Autodesk Fusion 360 part; units mm, degrees
(part 3 of 7)
  spline S37 degree 5 poles (-31.8463, 21.6348) (-31.8387, 21.6182) (-31.8236, 21.585) (-31.8007, 21.5353) (-31.7701, 21.4693) (-31.7314, 21.387) (-31.6925, 21.3049) (-31.6532, 21.2232) (-31.6135, 21.1418) (-31.5736, 21.0606) (-31.5333, 20.9798) (-31.4926, 20.8992) (-31.4516, 20.8189) (-31.4103, 20.739) (-31.3687, 20.6594) (-31.3267, 20.58) (-31.2844, 20.501) (-31.2417, 20.4223) (-31.1987, 20.3439) (-31.1553, 20.2659) (-31.1116, 20.1882) (-31.0676, 20.1108) (-31.0232, 20.0337) (-30.9785, 19.957) (-30.9334, 19.8806) (-30.888, 19.8046) (-30.8422, 19.7289) (-30.796, 19.6536) (-30.7496, 19.5787) (-30.7027, 19.5041) (-30.6555, 19.4299) (-30.608, 19.356) (-30.5601, 19.2825) (-30.5118, 19.2094) (-30.4631, 19.1368) (-30.4141, 19.0645) (-30.3647, 18.9925) (-30.315, 18.921) (-30.2649, 18.85) (-30.2144, 18.7793) (-30.1635, 18.709) (-30.1123, 18.6392) (-30.0606, 18.5699) (-30.0086, 18.5009) (-29.9561, 18.4325) (-29.9033, 18.3645) (-29.8501, 18.297) (-29.7965, 18.2299) (-29.7425, 18.1633) (-29.6881, 18.0972) (-29.6333, 18.0316) (-29.578, 17.9666) (-29.5222, 17.9021) (-29.466, 17.8383) (-29.4094, 17.775) (-29.3523, 17.7122) (-29.2948, 17.65) (-29.2369, 17.5883) (-29.1786, 17.5272) (-29.1198, 17.4666) (-29.0604, 17.4069) (-29.0004, 17.348) (-28.9396, 17.2901) (-28.8782, 17.2332) (-28.8162, 17.1772) (-28.7537, 17.1217) (-28.6909, 17.0668) (-28.6278, 17.0123) (-28.5642, 16.9585) (-28.4998, 16.906) (-28.434, 16.8556) (-28.3799, 16.8175) (-28.3382, 16.7905) (-28.3099, 16.7732) (-28.2957, 16.7647) knots -1 -1 -1 -1 -1 -1 -0.98571429 -0.97142857 -0.95714286 -0.94285714 -0.92857143 -0.91428571 -0.9 -0.88571429 -0.87142857 -0.85714286 -0.84285714 -0.82857143 -0.81428571 -0.8 -0.78571429 -0.77142857 -0.75714286 -0.74285714 -0.72857143 -0.71428571 -0.7 -0.68571429 -0.67142857 -0.65714286 -0.64285714 -0.62857143 -0.61428571 -0.6 -0.58571429 -0.57142857 -0.55714286 -0.54285714 -0.52857143 -0.51428571 -0.5 -0.48571429 -0.47142857 -0.45714286 -0.44285714 -0.42857143 -0.41428571 -0.4 -0.38571429 -0.37142857 -0.35714286 -0.34285714 -0.32857143 -0.31428571 -0.3 -0.28571429 -0.27142857 -0.25714286 -0.24285714 -0.22857143 -0.21428571 -0.2 -0.18571429 -0.17142857 -0.15714286 -0.14285714 -0.12857143 -0.11428571 -0.1 -0.08571429 -0.07142857 -0.05714286 -0.04285714 -0.02857143 -0.01428571 0 0 0 0 0 0
  line L37 (-28.2957, 16.7647) -> (-27.7863, 16.4626)
  arc A75 (-27.1922, 14.356) -> (-27.7863, 16.4626) centre (-28.5961, 15.0972) ccw
  arc A76 (-27.1922, 14.356) -> (-27.5975, 13.5607) centre (0, 0) ccw
  arc A77 (-29.6509, 12.8031) -> (-27.5975, 13.5607) centre (-29.0223, 14.2608) ccw
  line L38 (-29.6509, 12.8031) -> (-30.1947, 13.0376)
  spline S38 degree 5 poles (-30.1947, 13.0376) (-30.21, 13.0442) (-30.2406, 13.0569) (-30.2869, 13.0748) (-30.3496, 13.0962) (-30.429, 13.1197) (-30.5094, 13.141) (-30.5903, 13.1608) (-30.6714, 13.1798) (-30.7528, 13.1984) (-30.8344, 13.2163) (-30.9162, 13.2335) (-30.9983, 13.2498) (-31.0808, 13.2649) (-31.1637, 13.2788) (-31.247, 13.2917) (-31.3305, 13.3037) (-31.4142, 13.315) (-31.4982, 13.3255) (-31.5823, 13.3355) (-31.6666, 13.3448) (-31.7511, 13.3534) (-31.8359, 13.3614) (-31.9208, 13.3686) (-32.0059, 13.3751) (-32.0911, 13.3809) (-32.1766, 13.3861) (-32.2622, 13.3906) (-32.348, 13.3946) (-32.4339, 13.3979) (-32.52, 13.4007) (-32.6062, 13.4029) (-32.6925, 13.4045) (-32.779, 13.4055) (-32.8656, 13.4059) (-32.9523, 13.4058) (-33.0392, 13.4051) (-33.1262, 13.4038) (-33.2132, 13.4021) (-33.3004, 13.3997) (-33.3877, 13.3969) (-33.4751, 13.3935) (-33.5626, 13.3896) (-33.6502, 13.3852) (-33.7379, 13.3803) (-33.8257, 13.3748) (-33.9136, 13.3689) (-34.0016, 13.3624) (-34.0896, 13.3555) (-34.1778, 13.348) (-34.266, 13.3401) (-34.3542, 13.3317) (-34.4426, 13.3228) (-34.531, 13.3134) (-34.6195, 13.3035) (-34.7081, 13.2932) (-34.7967, 13.2824) (-34.8854, 13.2711) (-34.9741, 13.2594) (-35.063, 13.2472) (-35.1518, 13.2345) (-35.2407, 13.2214) (-35.3297, 13.2078) (-35.4187, 13.1938) (-35.5078, 13.1793) (-35.5969, 13.1644) (-35.686, 13.1491) (-35.7752, 13.1333) (-35.8644, 13.117) (-35.9537, 13.1003) (-36.043, 13.0832) (-36.1145, 13.0692) (-36.1681, 13.0584) (-36.2038, 13.0512) (-36.2217, 13.0476) knots 0 0 0 0 0 0 0.01428571 0.02857143 0.04285714 0.05714286 0.07142857 0.08571429 0.1 0.11428571 0.12857143 0.14285714 0.15714286 0.17142857 0.18571429 0.2 0.21428571 0.22857143 0.24285714 0.25714286 0.27142857 0.28571429 0.3 0.31428571 0.32857143 0.34285714 0.35714286 0.37142857 0.38571429 0.4 0.41428571 0.42857143 0.44285714 0.45714286 0.47142857 0.48571429 0.5 0.51428571 0.52857143 0.54285714 0.55714286 0.57142857 0.58571429 0.6 0.61428571 0.62857143 0.64285714 0.65714286 0.67142857 0.68571429 0.7 0.71428571 0.72857143 0.74285714 0.75714286 0.77142857 0.78571429 0.8 0.81428571 0.82857143 0.84285714 0.85714286 0.87142857 0.88571429 0.9 0.91428571 0.92857143 0.94285714 0.95714286 0.97142857 0.98571429 1 1 1 1 1 1
  arc A78 (-36.2217, 13.0476) -> (-36.9731, 10.7349) centre (0, 0) ccw
  spline S39 degree 5 poles (-36.9731, 10.7349) (-36.9608, 10.7214) (-36.9361, 10.6946) (-36.8991, 10.6544) (-36.8495, 10.601) (-36.7873, 10.5347) (-36.7249, 10.4687) (-36.6623, 10.4031) (-36.5994, 10.3379) (-36.5363, 10.2731) (-36.473, 10.2086) (-36.4095, 10.1446) (-36.3457, 10.0809) (-36.2817, 10.0176) (-36.2175, 9.9548) (-36.153, 9.8923) (-36.0883, 9.8302) (-36.0235, 9.7686) (-35.9583, 9.7073) (-35.893, 9.6465) (-35.8274, 9.5861) (-35.7616, 9.5261) (-35.6956, 9.4665) (-35.6293, 9.4074) (-35.5629, 9.3487) (-35.4962, 9.2904) (-35.4292, 9.2326) (-35.3621, 9.1752) (-35.2947, 9.1183) (-35.2271, 9.0618) (-35.1593, 9.0058) (-35.0912, 8.9503) (-35.023, 8.8952) (-34.9545, 8.8406) (-34.8857, 8.7865) (-34.8168, 8.7329) (-34.7476, 8.6798) (-34.6782, 8.6271) (-34.6086, 8.575) (-34.5387, 8.5234) (-34.4686, 8.4723) (-34.3983, 8.4218) (-34.3277, 8.3717) (-34.257, 8.3223) (-34.1859, 8.2734) (-34.1147, 8.225) (-34.0432, 8.1773) (-33.9715, 8.13) (-33.8996, 8.0834) (-33.8274, 8.0373) (-33.755, 7.9919) (-33.6823, 7.9471) (-33.6094, 7.9031) (-33.5362, 7.8597) (-33.4627, 7.817) (-33.389, 7.775) (-33.3151, 7.7336) (-33.241, 7.6928) (-33.1666, 7.6526) (-33.092, 7.6133) (-33.0171, 7.5748) (-32.9418, 7.5373) (-32.8662, 7.5011) (-32.7902, 7.4659) (-32.7139, 7.4318) (-32.6373, 7.3983) (-32.5606, 7.3655) (-32.4838, 7.3332) (-32.4067, 7.3017) (-32.3292, 7.2716) (-32.251, 7.244) (-32.1878, 7.2245) (-32.1398, 7.2117) (-32.1076, 7.204) (-32.0914, 7.2004) knots -1 -1 -1 -1 -1 -1 -0.98571429 -0.97142857 -0.95714286 -0.94285714 -0.92857143 -0.91428571 -0.9 -0.88571429 -0.87142857 -0.85714286 -0.84285714 -0.82857143 -0.81428571 -0.8 -0.78571429 -0.77142857 -0.75714286 -0.74285714 -0.72857143 -0.71428571 -0.7 -0.68571429 -0.67142857 -0.65714286 -0.64285714 -0.62857143 -0.61428571 -0.6 -0.58571429 -0.57142857 -0.55714286 -0.54285714 -0.52857143 -0.51428571 -0.5 -0.48571429 -0.47142857 -0.45714286 -0.44285714 -0.42857143 -0.41428571 -0.4 -0.38571429 -0.37142857 -0.35714286 -0.34285714 -0.32857143 -0.31428571 -0.3 -0.28571429 -0.27142857 -0.25714286 -0.24285714 -0.22857143 -0.21428571 -0.2 -0.18571429 -0.17142857 -0.15714286 -0.14285714 -0.12857143 -0.11428571 -0.1 -0.08571429 -0.07142857 -0.05714286 -0.04285714 -0.02857143 -0.01428571 0 0 0 0 0 0
  line L39 (-32.0914, 7.2004) -> (-31.5136, 7.0705)
  arc A79 (-30.2976, 5.2505) -> (-31.5136, 7.0705) centre (-31.8618, 5.5216) ccw
  circle A80 centre (0, 0) radius 7.5
  dimension "d9" = 15
  constraint coincident A0.centre A2.centre
  measures "d9" diameter of A80
extrude "Extruir3" add sketch "Boceto2 (2)" along normal blind 50 contours A80 bodies 1 in component "Spur Gear (20 teeth)"
sketch "Boceto3 (2)" plane through (0, 0, 63) normal (0, 0, 1) x (-1, 0, 0)
  circle A0 centre (0, 0) radius 7.5
  circle A1 centre (0, 0) radius 7.5
  constraint coincident A0.centre A1.centre
extrude "Extruir4" add sketch "Boceto3 (2)" along normal blind 15.297 bodies 1 in component "Spur Gear (20 teeth)"
sketch "Boceto4" plane through (0, 0, 78.297) normal (0, 0, 1) x (-1, 0, 0)
  circle A0 centre (0, 0) radius 7.5
  circle A1 centre (0, 0) radius 15
  dimension "d14" = 30
  constraint concentric A0 A1
  measures "d14" diameter of A1
extrude "Extruir1'" add sketch "Boceto4" along normal blind 2 separate body makes body 2
sketch "Boceto5" plane through (0, 0, 78.297) normal (0, 0, 1) x (-1, 0, 0)
  circle A0 centre (0, 0) radius 7.5
  circle A1 centre (0, 0) radius 7.5
  constraint coincident A0.centre A1.centre
extrude "Extruir2'" add sketch "Boceto5" along normal blind 2 bodies 2
sketch "Boceto6" plane through (0, 0, 80.297) normal (0, 0, 1) x (-1, 0, 0)
  circle A0 centre (0, 0) radius 15
  circle A1 centre (0, 12) radius 1
  circle A2 centre (-12, 0) radius 1
  circle A3 centre (12, 0) radius 1
  circle A4 centre (0, -12) radius 1
  dimension "d19" = 12
  dimension "d20" = 12
  dimension "d21" = 12
  dimension "d22" = 12
  dimension "d23" = 2
  dimension "d24" = 2
  dimension "d25" = 2
  dimension "d26" = 2
  measures "d19" distance of A0.centre A1.centre
  measures "d20" distance of A0.centre A2.centre
  measures "d21" distance of A0.centre A4.centre
  measures "d22" distance of A0.centre A3.centre
  measures "d23" diameter of A1
  measures "d24" diameter of A2
  measures "d25" diameter of A4
  measures "d26" diameter of A3
extrude "Extruir3'" cut sketch "Boceto6" against normal blind 2 contours A1 | A2 | A3 | A4 bodies 2
component "Spur Gear (20 teeth)" placed x (1, 0, 0) y (0, 1, 0) z (0, 0, 1) at (0, 0, 0)

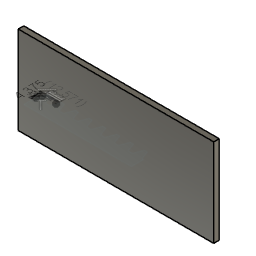
design "puerta mecatronica"
Autodesk Fusion 360 part; units mm, degrees
sketch "Boceto1" plane through (0, 0, 0) normal (0, 0, 1) x (1, 0, 0)
  line L0 (0, 0) -> (2.8663, 7.875)
  line L1 (0, 0) -> (64.0312, 0) construction
  line L2 (0, 0) -> (0, 4.375) construction
  line L3 (0, 4.375) -> (1.5924, 4.375) construction
  line L4 (1.5924, 4.375) -> (7.0924, 4.375) construction
  line L5 (7.0924, 4.375) -> (8.6847, 0)
  line L6 (7.0924, 4.375) -> (12.0861, 4.375) construction
  line L7 (7.0924, 4.375) -> (5.8185, 7.875)
  line L8 (7.0924, 4.375) -> (11.3868, 4.375) construction
  line L9 (5.8185, 7.875) -> (2.8663, 7.875)
  line L10 (8.6847, 0) -> (0, 0)
  dimension "d1" = 70
  dimension "d2" = 7.875
  dimension "d3" = 4.375
  dimension "d4" = 5.5
  dimension "d5" = 70
  dimension "d6" = 4.375
  dimension "d7" = 110
  dimension "d8" = 3.5
  constraint horizontal L1
  constraint coincident L0.start L1.start
  constraint perpendicular L1 L2
  constraint coincident L0 L3.end
  constraint perpendicular L2 L3
  constraint perpendicular L2 L4
  constraint horizontal L6
  constraint horizontal L8
  measures "d1" angle of L0 L1
  measures "d2" distance of L0.start L0.end
  measures "d3" distance of L0.start L2.end
  measures "d4" distance of L3.end L4.end
  measures "d5" angle of L5 L6
  measures "d6" distance of L4.end L5.end
  measures "d7" angle of L7 L8
  measures "d8" distance of L4.end L7.end
extrude "Extruir1" add sketch "Boceto1" along normal blind 13 makes body 1
pattern_linear "Patrón R1" count 8 spacing 12.5714 along (1, 0, 0) of "Extruir1" makes body 2 at (15.4663, 0, 8.6667) makes body 3 at (30.9327, 0, 8.6667) makes body 4 at (43.5041, 0, 4.3333) makes body 5 at (56.0755, 0, 4.3333) makes body 6 at (68.647, 0, 8.6667) makes body 7 at (81.2184, 0, 4.3333) makes body 8 at (93.7898, 0, 4.3333)
sketch "Boceto2" plane through (0, 0, 13) normal (0, 0, 1) x (-1, 0, 0)
  line L0 (-8.6847, 0) -> (-5.8185, -7.875)
  line L1 (-5.8185, -7.875) -> (-2.8663, -7.875)
  line L2 (-2.8663, -7.875) -> (0, 0)
  line L3 (0, 0) -> (-8.6847, 0)
  line L4 (0, 0) -> (-98, 0)
  line L5 (-98, 0) -> (-98, 16)
  line L6 (-98, 16) -> (0, 16)
  line L7 (0, 16) -> (0, 0)
  constraint horizontal L4
  constraint vertical L5
  constraint horizontal L6
  constraint vertical L7
  constraint coincident L2.end L3.start
extrude "Extruir2" add sketch "Boceto2" against normal blind 13 contours L3 L4 L5 L6 L7 bodies 1 2 3 4 5 6 7 8
fillet "Empalme1" radius 1.05 15 edges at (8.6847, 0, 6.5) (12.5714, 0, 6.5) (21.2562, 0, 6.5) (25.1429, 0, 6.5) (33.8276, 0, 6.5) (37.7143, 0, 6.5) (46.399, 0, 6.5) (50.2857, 0, 6.5) (58.9705, 0, 6.5) (62.8571, 0, 6.5) (71.5419, 0, 6.5) (75.4286, 0, 6.5) (84.1133, 0, 6.5) (88, 0, 6.5) (96.6847, 0, 6.5) on bodies 1
sketch "Boceto3" plane through (0, 0, 13) normal (0, 0, 1) x (-1, 0, 0)
  line L0 (-83.8619, -0.6909) -> (-81.247, -7.875)
  line L1 (-81.247, -7.875) -> (-78.2948, -7.875)
  line L2 (-78.2948, -7.875) -> (-75.68, -0.6909)
  arc A0 (-74.6934, 0) -> (-75.68, -0.6909) centre (-74.6934, -1.05) ccw
  line L3 (-74.6934, 0) -> (-72.2771, 0)
  arc A1 (-71.2904, -0.6909) -> (-72.2771, 0) centre (-72.2771, -1.05) ccw
  line L4 (-71.2904, -0.6909) -> (-68.6756, -7.875)
  line L5 (-68.6756, -7.875) -> (-65.7234, -7.875)
  line L6 (-65.7234, -7.875) -> (-63.1086, -0.6909)
  arc A2 (-62.1219, 0) -> (-63.1086, -0.6909) centre (-62.1219, -1.05) ccw
  line L7 (-62.1219, 0) -> (-59.7057, 0)
  arc A3 (-58.719, -0.6909) -> (-59.7057, 0) centre (-59.7057, -1.05) ccw
  line L8 (-58.719, -0.6909) -> (-56.1042, -7.875)
  line L9 (-56.1042, -7.875) -> (-53.152, -7.875)
  line L10 (-53.152, -7.875) -> (-50.5372, -0.6909)
  arc A4 (-49.5505, 0) -> (-50.5372, -0.6909) centre (-49.5505, -1.05) ccw
  line L11 (-49.5505, 0) -> (-47.1342, 0)
  arc A5 (-46.1476, -0.6909) -> (-47.1342, 0) centre (-47.1342, -1.05) ccw
  line L12 (-46.1476, -0.6909) -> (-43.5328, -7.875)
  line L13 (-43.5328, -7.875) -> (-40.5806, -7.875)
  line L14 (-40.5806, -7.875) -> (-37.9657, -0.6909)
  arc A6 (-36.9791, 0) -> (-37.9657, -0.6909) centre (-36.9791, -1.05) ccw
  line L15 (-36.9791, 0) -> (-34.5628, 0)
  arc A7 (-33.5761, -0.6909) -> (-34.5628, 0) centre (-34.5628, -1.05) ccw
  line L16 (-33.5761, -0.6909) -> (-30.9613, -7.875)
  line L17 (-30.9613, -7.875) -> (-28.0091, -7.875)
  line L18 (-28.0091, -7.875) -> (-25.3943, -0.6909)
  arc A8 (-24.4076, 0) -> (-25.3943, -0.6909) centre (-24.4076, -1.05) ccw
  line L19 (-24.4076, 0) -> (-21.9914, 0)
  arc A9 (-21.0047, -0.6909) -> (-21.9914, 0) centre (-21.9914, -1.05) ccw
  line L20 (-21.0047, -0.6909) -> (-18.3899, -7.875)
  line L21 (-18.3899, -7.875) -> (-15.4377, -7.875)
  line L22 (-15.4377, -7.875) -> (-12.8229, -0.6909)
  arc A10 (-11.8362, 0) -> (-12.8229, -0.6909) centre (-11.8362, -1.05) ccw
  line L23 (-11.8362, 0) -> (-9.42, 0)
  arc A11 (-8.4333, -0.6909) -> (-9.42, 0) centre (-9.42, -1.05) ccw
  line L24 (-8.4333, -0.6909) -> (-5.8185, -7.875)
  line L25 (-5.8185, -7.875) -> (-2.8663, -7.875)
  line L26 (-2.8663, -7.875) -> (0, 0)
  line L27 (0, 0) -> (0, 16)
  line L28 (0, 16) -> (-98, 16)
  line L29 (-98, 16) -> (-98, 0)
  line L30 (-98, 0) -> (-97.42, 0)
  arc A12 (-96.4333, -0.6909) -> (-97.42, 0) centre (-97.42, -1.05) ccw
  line L31 (-96.4333, -0.6909) -> (-93.8185, -7.875)
  line L32 (-93.8185, -7.875) -> (-90.8663, -7.875)
  line L33 (-90.8663, -7.875) -> (-88.2515, -0.6909)
  arc A13 (-87.2648, 0) -> (-88.2515, -0.6909) centre (-87.2648, -1.05) ccw
  line L34 (-87.2648, 0) -> (-84.8485, 0)
  arc A14 (-83.8619, -0.6909) -> (-84.8485, 0) centre (-84.8485, -1.05) ccw
  line L35 (0, 16) -> (-98, 16)
  line L36 (-98, 16) -> (-98, 11)
  line L37 (-98, 11) -> (0, 11)
  line L38 (0, 11) -> (0, 16)
  dimension "d19" = 5
  constraint horizontal L35
  constraint vertical L36
  constraint horizontal L37
  constraint vertical L38
  constraint coincident L29 L36.end
  constraint coincident L27.end L28.start
  measures "d19" distance of L27.end L37.end
extrude "Extruir3" add sketch "Boceto3" along normal blind 30 contours L27 L28 L29 L35 L36 L37 L38 bodies 1
sketch "Boceto4" plane through (0, 0, 0) normal (1, 0, 0) x (0, 1, 0)
sketch "Boceto5" plane through (0, 0, 0) normal (0, 0, -1) x (1, 0, 0)
  arc A0 (84.8485, 0) -> (83.8619, -0.6909) centre (84.8485, -1.05) ccw
  line L0 (84.8485, 0) -> (87.2648, 0)
  arc A1 (88.2515, -0.6909) -> (87.2648, 0) centre (87.2648, -1.05) ccw
  line L1 (88.2515, -0.6909) -> (90.8663, -7.875)
  line L2 (90.8663, -7.875) -> (93.8185, -7.875)
  line L3 (93.8185, -7.875) -> (96.4333, -0.6909)
  arc A2 (97.42, 0) -> (96.4333, -0.6909) centre (97.42, -1.05) ccw
  line L4 (97.42, 0) -> (98, 0)
  line L5 (98, 0) -> (98, 16)
  line L6 (98, 16) -> (0, 16)
  line L7 (0, 16) -> (0, 0)
  line L8 (0, 0) -> (2.8663, -7.875)
  line L9 (2.8663, -7.875) -> (5.8185, -7.875)
  line L10 (5.8185, -7.875) -> (8.4333, -0.6909)
  arc A3 (9.42, 0) -> (8.4333, -0.6909) centre (9.42, -1.05) ccw
  line L11 (9.42, 0) -> (11.8362, 0)
  arc A4 (12.8229, -0.6909) -> (11.8362, 0) centre (11.8362, -1.05) ccw
  line L12 (12.8229, -0.6909) -> (15.4377, -7.875)
  line L13 (15.4377, -7.875) -> (18.3899, -7.875)
  line L14 (18.3899, -7.875) -> (21.0047, -0.6909)
  arc A5 (21.9914, 0) -> (21.0047, -0.6909) centre (21.9914, -1.05) ccw
  line L15 (21.9914, 0) -> (24.4076, 0)
  arc A6 (25.3943, -0.6909) -> (24.4076, 0) centre (24.4076, -1.05) ccw
  line L16 (25.3943, -0.6909) -> (28.0091, -7.875)
  line L17 (28.0091, -7.875) -> (30.9613, -7.875)
  line L18 (30.9613, -7.875) -> (33.5761, -0.6909)
  arc A7 (34.5628, 0) -> (33.5761, -0.6909) centre (34.5628, -1.05) ccw
  line L19 (34.5628, 0) -> (36.9791, 0)
  arc A8 (37.9657, -0.6909) -> (36.9791, 0) centre (36.9791, -1.05) ccw
  line L20 (37.9657, -0.6909) -> (40.5806, -7.875)
  line L21 (40.5806, -7.875) -> (43.5328, -7.875)
  line L22 (43.5328, -7.875) -> (46.1476, -0.6909)
  arc A9 (47.1342, 0) -> (46.1476, -0.6909) centre (47.1342, -1.05) ccw
  line L23 (47.1342, 0) -> (49.5505, 0)
  arc A10 (50.5372, -0.6909) -> (49.5505, 0) centre (49.5505, -1.05) ccw
  line L24 (50.5372, -0.6909) -> (53.152, -7.875)
  line L25 (53.152, -7.875) -> (56.1042, -7.875)
  line L26 (56.1042, -7.875) -> (58.719, -0.6909)
  arc A11 (59.7057, 0) -> (58.719, -0.6909) centre (59.7057, -1.05) ccw
  line L27 (59.7057, 0) -> (62.1219, 0)
  arc A12 (63.1086, -0.6909) -> (62.1219, 0) centre (62.1219, -1.05) ccw
  line L28 (63.1086, -0.6909) -> (65.7234, -7.875)
  line L29 (65.7234, -7.875) -> (68.6756, -7.875)
  line L30 (68.6756, -7.875) -> (71.2904, -0.6909)
  arc A13 (72.2771, 0) -> (71.2904, -0.6909) centre (72.2771, -1.05) ccw
  line L31 (72.2771, 0) -> (74.6934, 0)
  arc A14 (75.68, -0.6909) -> (74.6934, 0) centre (74.6934, -1.05) ccw
  line L32 (75.68, -0.6909) -> (78.2948, -7.875)
  line L33 (78.2948, -7.875) -> (81.247, -7.875)
  line L34 (81.247, -7.875) -> (83.8619, -0.6909)
  line L35 (98, 16) -> (0, 16)
  line L36 (0, 16) -> (0, 11)
  line L37 (0, 11) -> (98, 11)
  line L38 (98, 11) -> (98, 16)
  constraint horizontal L35
  constraint vertical L36
  constraint horizontal L37
  constraint vertical L38
  constraint coincident L7 L36.end
  constraint coincident L5.end L6.start
extrude "Extruir4" add sketch "Boceto5" along normal blind 5 contours L5 L6 L7 L35 L36 L37 L38 bodies 1
sketch "Boceto6" plane through (0, 0, 43) normal (0, 0, 1) x (-1, 0, 0)
  line L0 (0, 11) -> (0, 16)
  line L1 (0, 16) -> (-98, 16)
  line L2 (-98, 16) -> (-98, 11)
  line L3 (-98, 11) -> (0, 11)
  line L4 (0, 16) -> (-98, 16)
  line L5 (-98, 16) -> (-98, 11)
  line L6 (-98, 11) -> (0, 11)
  line L7 (0, 11) -> (0, 16)
  constraint horizontal L4
  constraint vertical L5
  constraint horizontal L6
  constraint vertical L7
  constraint coincident L2.end L3.start
  constraint coincident L0.end L1.start
extrude "Extruir5" add sketch "Boceto6" along normal blind 32 bodies 1
sketch "Boceto7" plane through (98, 0, 0) normal (1, 0, 0) x (0, 1, 0)
  line L0 (0, 13) -> (-11, 13)
  line L1 (-11, 13) -> (-11, 75)
  line L2 (-11, 75) -> (-16, 75)
  line L3 (-16, 75) -> (-16, -5)
  line L4 (-16, -5) -> (-11, -5)
  line L5 (-11, -5) -> (-11, 0)
  line L6 (-11, 0) -> (0, 0)
  line L7 (0, 0) -> (0, 13)
  line L8 (-11, 75) -> (-16, 75)
  line L9 (-16, 75) -> (-16, -5)
  line L10 (-16, -5) -> (-11, -5)
  line L11 (-11, -5) -> (-11, 75)
  constraint horizontal L8
  constraint vertical L9
  constraint horizontal L10
  constraint vertical L11
  constraint coincident L3.end L4.start
  constraint coincident L1.end L2.start
extrude "Extruir6" add sketch "Boceto7" along normal blind 80 contours L1 L2 L3 L4 L5 L8 L9 L10 L11 bodies 1
sketch "Boceto8" plane through (0, 0, 13) normal (0, 0, 1) x (-1, 0, 0)
  line L0 (0, 11) -> (-98, 11)
  line L1 (-98, 11) -> (-98, 0)
  line L2 (-98, 0) -> (-97.42, 0)
  arc A0 (-96.4333, -0.6909) -> (-97.42, 0) centre (-97.42, -1.05) ccw
  line L3 (-96.4333, -0.6909) -> (-93.8185, -7.875)
  line L4 (-93.8185, -7.875) -> (-90.8663, -7.875)
  line L5 (-90.8663, -7.875) -> (-88.2515, -0.6909)
  arc A1 (-87.2648, 0) -> (-88.2515, -0.6909) centre (-87.2648, -1.05) ccw
  line L6 (-87.2648, 0) -> (-84.8485, 0)
  arc A2 (-83.8619, -0.6909) -> (-84.8485, 0) centre (-84.8485, -1.05) ccw
  line L7 (-83.8619, -0.6909) -> (-81.247, -7.875)
  line L8 (-81.247, -7.875) -> (-78.2948, -7.875)
  line L9 (-78.2948, -7.875) -> (-75.68, -0.6909)
  arc A3 (-74.6934, 0) -> (-75.68, -0.6909) centre (-74.6934, -1.05) ccw
  line L10 (-74.6934, 0) -> (-72.2771, 0)
  arc A4 (-71.2904, -0.6909) -> (-72.2771, 0) centre (-72.2771, -1.05) ccw
  line L11 (-71.2904, -0.6909) -> (-68.6756, -7.875)
  line L12 (-68.6756, -7.875) -> (-65.7234, -7.875)
  line L13 (-65.7234, -7.875) -> (-63.1086, -0.6909)
  arc A5 (-62.1219, 0) -> (-63.1086, -0.6909) centre (-62.1219, -1.05) ccw
  line L14 (-62.1219, 0) -> (-59.7057, 0)
  arc A6 (-58.719, -0.6909) -> (-59.7057, 0) centre (-59.7057, -1.05) ccw
  line L15 (-58.719, -0.6909) -> (-56.1042, -7.875)
  line L16 (-56.1042, -7.875) -> (-53.152, -7.875)
  line L17 (-53.152, -7.875) -> (-50.5372, -0.6909)
  arc A7 (-49.5505, 0) -> (-50.5372, -0.6909) centre (-49.5505, -1.05) ccw
  line L18 (-49.5505, 0) -> (-47.1342, 0)
  arc A8 (-46.1476, -0.6909) -> (-47.1342, 0) centre (-47.1342, -1.05) ccw
  line L19 (-46.1476, -0.6909) -> (-43.5328, -7.875)
  line L20 (-43.5328, -7.875) -> (-40.5806, -7.875)
  line L21 (-40.5806, -7.875) -> (-37.9657, -0.6909)
  arc A9 (-36.9791, 0) -> (-37.9657, -0.6909) centre (-36.9791, -1.05) ccw
  line L22 (-36.9791, 0) -> (-34.5628, 0)
  arc A10 (-33.5761, -0.6909) -> (-34.5628, 0) centre (-34.5628, -1.05) ccw
  line L23 (-33.5761, -0.6909) -> (-30.9613, -7.875)
  line L24 (-30.9613, -7.875) -> (-28.0091, -7.875)
  line L25 (-28.0091, -7.875) -> (-25.3943, -0.6909)
  arc A11 (-24.4076, 0) -> (-25.3943, -0.6909) centre (-24.4076, -1.05) ccw
  line L26 (-24.4076, 0) -> (-21.9914, 0)
  arc A12 (-21.0047, -0.6909) -> (-21.9914, 0) centre (-21.9914, -1.05) ccw
  line L27 (-21.0047, -0.6909) -> (-18.3899, -7.875)
  line L28 (-18.3899, -7.875) -> (-15.4377, -7.875)
  line L29 (-15.4377, -7.875) -> (-12.8229, -0.6909)
  arc A13 (-11.8362, 0) -> (-12.8229, -0.6909) centre (-11.8362, -1.05) ccw
  line L30 (-11.8362, 0) -> (-9.42, 0)
  arc A14 (-8.4333, -0.6909) -> (-9.42, 0) centre (-9.42, -1.05) ccw
  line L31 (-8.4333, -0.6909) -> (-5.8185, -7.875)
  line L32 (-5.8185, -7.875) -> (-2.8663, -7.875)
  line L33 (-2.8663, -7.875) -> (0, 0)
  line L34 (0, 0) -> (0, 11)
  line L35 (0, 0) -> (0, -4.375) construction
  line L36 (0, -4.375) -> (-1.5924, -4.375) construction
  line L37 (-1.5924, -4.375) -> (-14.1638, -4.375) construction
  dimension "d28" = 4.375
  dimension "d29" = 12.5714
  constraint coincident L33.end L34.start
  constraint parallel L34 L35
  constraint coincident L33 L36.end
  constraint perpendicular L35 L36
  constraint coincident L29 L37.end
  constraint horizontal L37
  measures "d28" distance of L33.end L35.end
  measures "d29" distance of L36.end L37.end

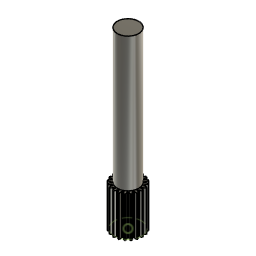
design "engranaje mecatronica"
part number: arrangementsContainer
description: Spur Gear; Module: 0.5; Num Teeth: 20; Pressure Angle: 20.0; Backlash: 0.00 mm
Autodesk Fusion 360 part; units mm, degrees
sketch "Boceto1" plane through (0, 0, 0) normal (0, 0, 1) x (1, 0, 0) in component "Spur Gear (20 teeth)"
  circle A0 centre (0, 0) radius 4.3492
extrude "Extruir1" add sketch "Boceto1" along normal blind 15 in component "Spur Gear (20 teeth)"
sketch "Boceto2" plane through (0, 0, 0) normal (0, 0, 1) x (1, 0, 0) in component "Spur Gear (20 teeth)"
  spline S0 degree 5 poles (4.678, -0.4384) (4.6803, -0.4386) (4.6849, -0.439) (4.6919, -0.4393) (4.7012, -0.4395) (4.7128, -0.4392) (4.7245, -0.4386) (4.7361, -0.4378) (4.7478, -0.4368) (4.7595, -0.4357) (4.7712, -0.4346) (4.7829, -0.4334) (4.7947, -0.432) (4.8064, -0.4304) (4.8181, -0.4287) (4.8299, -0.4269) (4.8416, -0.4248) (4.8534, -0.4227) (4.8651, -0.4205) (4.8769, -0.4182) (4.8886, -0.4158) (4.9004, -0.4133) (4.9122, -0.4106) (4.9239, -0.4079) (4.9357, -0.4051) (4.9475, -0.4022) (4.9593, -0.3991) (4.971, -0.396) (4.9828, -0.3928) (4.9946, -0.3895) (5.0064, -0.3861) (5.0181, -0.3826) (5.0299, -0.3791) (5.0417, -0.3754) (5.0535, -0.3717) (5.0652, -0.3679) (5.077, -0.364) (5.0888, -0.36) (5.1005, -0.3559) (5.1123, -0.3518) (5.124, -0.3476) (5.1358, -0.3433) (5.1475, -0.3389) (5.1593, -0.3344) (5.171, -0.3299) (5.1828, -0.3253) (5.1945, -0.3206) (5.2062, -0.3158) (5.2179, -0.311) (5.2297, -0.3061) (5.2414, -0.3011) (5.2531, -0.296) (5.2648, -0.2909) (5.2765, -0.2857) (5.2882, -0.2804) (5.2998, -0.2751) (5.3115, -0.2697) (5.3232, -0.2642) (5.3348, -0.2586) (5.3465, -0.253) (5.3581, -0.2473) (5.3698, -0.2415) (5.3814, -0.2357) (5.393, -0.2298) (5.4047, -0.2238) (5.4163, -0.2178) (5.4279, -0.2117) (5.4395, -0.2055) (5.451, -0.1993) (5.4626, -0.193) (5.4742, -0.1866) (5.4834, -0.1815) (5.4903, -0.1776) (5.4949, -0.175) (5.4973, -0.1737) knots 0 0 0 0 0 0 0.01428571 0.02857143 0.04285714 0.05714286 0.07142857 0.08571429 0.1 0.11428571 0.12857143 0.14285714 0.15714286 0.17142857 0.18571429 0.2 0.21428571 0.22857143 0.24285714 0.25714286 0.27142857 0.28571429 0.3 0.31428571 0.32857143 0.34285714 0.35714286 0.37142857 0.38571429 0.4 0.41428571 0.42857143 0.44285714 0.45714286 0.47142857 0.48571429 0.5 0.51428571 0.52857143 0.54285714 0.55714286 0.57142857 0.58571429 0.6 0.61428571 0.62857143 0.64285714 0.65714286 0.67142857 0.68571429 0.7 0.71428571 0.72857143 0.74285714 0.75714286 0.77142857 0.78571429 0.8 0.81428571 0.82857143 0.84285714 0.85714286 0.87142857 0.88571429 0.9 0.91428571 0.92857143 0.94285714 0.95714286 0.97142857 0.98571429 1 1 1 1 1 1
  spline S1 degree 5 poles (4.678, 0.4384) (4.6803, 0.4386) (4.6849, 0.439) (4.6919, 0.4393) (4.7012, 0.4395) (4.7128, 0.4392) (4.7245, 0.4386) (4.7361, 0.4378) (4.7478, 0.4368) (4.7595, 0.4357) (4.7712, 0.4346) (4.7829, 0.4334) (4.7947, 0.432) (4.8064, 0.4304) (4.8181, 0.4287) (4.8299, 0.4269) (4.8416, 0.4248) (4.8534, 0.4227) (4.8651, 0.4205) (4.8769, 0.4182) (4.8886, 0.4158) (4.9004, 0.4133) (4.9122, 0.4106) (4.9239, 0.4079) (4.9357, 0.4051) (4.9475, 0.4022) (4.9593, 0.3991) (4.971, 0.396) (4.9828, 0.3928) (4.9946, 0.3895) (5.0064, 0.3861) (5.0181, 0.3826) (5.0299, 0.3791) (5.0417, 0.3754) (5.0535, 0.3717) (5.0652, 0.3679) (5.077, 0.364) (5.0888, 0.36) (5.1005, 0.3559) (5.1123, 0.3518) (5.124, 0.3476) (5.1358, 0.3433) (5.1475, 0.3389) (5.1593, 0.3344) (5.171, 0.3299) (5.1828, 0.3253) (5.1945, 0.3206) (5.2062, 0.3158) (5.2179, 0.311) (5.2297, 0.3061) (5.2414, 0.3011) (5.2531, 0.296) (5.2648, 0.2909) (5.2765, 0.2857) (5.2882, 0.2804) (5.2998, 0.2751) (5.3115, 0.2697) (5.3232, 0.2642) (5.3348, 0.2586) (5.3465, 0.253) (5.3581, 0.2473) (5.3698, 0.2415) (5.3814, 0.2357) (5.393, 0.2298) (5.4047, 0.2238) (5.4163, 0.2178) (5.4279, 0.2117) (5.4395, 0.2055) (5.451, 0.1993) (5.4626, 0.193) (5.4742, 0.1866) (5.4834, 0.1815) (5.4903, 0.1776) (5.4949, 0.175) (5.4973, 0.1737) knots 0 0 0 0 0 0 0.01428571 0.02857143 0.04285714 0.05714286 0.07142857 0.08571429 0.1 0.11428571 0.12857143 0.14285714 0.15714286 0.17142857 0.18571429 0.2 0.21428571 0.22857143 0.24285714 0.25714286 0.27142857 0.28571429 0.3 0.31428571 0.32857143 0.34285714 0.35714286 0.37142857 0.38571429 0.4 0.41428571 0.42857143 0.44285714 0.45714286 0.47142857 0.48571429 0.5 0.51428571 0.52857143 0.54285714 0.55714286 0.57142857 0.58571429 0.6 0.61428571 0.62857143 0.64285714 0.65714286 0.67142857 0.68571429 0.7 0.71428571 0.72857143 0.74285714 0.75714286 0.77142857 0.78571429 0.8 0.81428571 0.82857143 0.84285714 0.85714286 0.87142857 0.88571429 0.9 0.91428571 0.92857143 0.94285714 0.95714286 0.97142857 0.98571429 1 1 1 1 1 1
  arc A0 (5.4973, -0.1737) -> (5.4973, 0.1737) centre (0, 0) ccw
  line L0 (4.3203, -0.4058) -> (4.678, -0.4384)
  line L1 (4.3203, 0.4058) -> (4.678, 0.4384)
  line L2 (4.3203, -0.4058) -> (4.3203, 0.4058)
  point P0 (4.7355, -0.4378)
  point P1 (4.7935, -0.4321)
  point P2 (4.8518, -0.423)
  point P3 (4.9103, -0.411)
  point P4 (4.9689, -0.3966)
  point P5 (5.0277, -0.3798)
  point P6 (5.0865, -0.3608)
  point P7 (5.1453, -0.3397)
  point P8 (5.2041, -0.3167)
  point P9 (5.2629, -0.2917)
  point P10 (5.3217, -0.2649)
  point P11 (5.3803, -0.2363)
  point P12 (5.4389, -0.2058)
  point P13 (4.7355, 0.4378)
  point P14 (4.7935, 0.4321)
  point P15 (4.8518, 0.423)
  point P16 (4.9103, 0.411)
  point P17 (4.9689, 0.3966)
  point P18 (5.0277, 0.3798)
  point P19 (5.0865, 0.3608)
  point P20 (5.1453, 0.3397)
  point P21 (5.2041, 0.3167)
  point P22 (5.2629, 0.2917)
  point P23 (5.3217, 0.2649)
  point P24 (5.3803, 0.2363)
  point P25 (5.4389, 0.2058)
extrude "Extruir2" add sketch "Boceto2" along normal blind 15 in component "Spur Gear (20 teeth)"
fillet "Empalme1" radius 0.1 2 edges at (4.3301, -0.4067, 7.5) (4.3301, 0.4067, 7.5) in component "Spur Gear (20 teeth)"
pattern_circular "Patrón C1" count 20 over 360 about axis through (0, 0, 0) along (0, 0, 1) of "Extruir2", "Empalme1" in component "Spur Gear (20 teeth)"
sketch "Boceto3" plane through (0, 0, 0) normal (0, 0, 1) x (1, 0, 0) in component "Spur Gear (20 teeth)"
  circle A0 centre (0, 0) radius 5 construction
sketch "Boceto1 (2)" plane through (0, 0, 15) normal (0, 0, 1) x (-1, 0, 0)
  arc A0 (-4.2641, 0.8559) -> (-4.3199, 0.5037) centre (0, 0) ccw
  arc A1 (-4.4283, 0.4157) -> (-4.3199, 0.5037) centre (-4.4193, 0.5152) ccw
  line L0 (-4.4283, 0.4157) -> (-4.678, 0.4384)
  spline S0 degree 5 poles (-4.678, 0.4384) (-4.6803, 0.4386) (-4.6849, 0.439) (-4.6919, 0.4393) (-4.7012, 0.4395) (-4.7128, 0.4392) (-4.7245, 0.4386) (-4.7361, 0.4378) (-4.7478, 0.4368) (-4.7595, 0.4357) (-4.7712, 0.4346) (-4.7829, 0.4334) (-4.7947, 0.432) (-4.8064, 0.4304) (-4.8181, 0.4287) (-4.8299, 0.4269) (-4.8416, 0.4248) (-4.8534, 0.4227) (-4.8651, 0.4205) (-4.8769, 0.4182) (-4.8886, 0.4158) (-4.9004, 0.4133) (-4.9122, 0.4106) (-4.9239, 0.4079) (-4.9357, 0.4051) (-4.9475, 0.4022) (-4.9593, 0.3991) (-4.971, 0.396) (-4.9828, 0.3928) (-4.9946, 0.3895) (-5.0064, 0.3861) (-5.0181, 0.3826) (-5.0299, 0.3791) (-5.0417, 0.3754) (-5.0535, 0.3717) (-5.0652, 0.3679) (-5.077, 0.364) (-5.0888, 0.36) (-5.1005, 0.3559) (-5.1123, 0.3518) (-5.124, 0.3476) (-5.1358, 0.3433) (-5.1475, 0.3389) (-5.1593, 0.3344) (-5.171, 0.3299) (-5.1828, 0.3253) (-5.1945, 0.3206) (-5.2062, 0.3158) (-5.2179, 0.311) (-5.2297, 0.3061) (-5.2414, 0.3011) (-5.2531, 0.296) (-5.2648, 0.2909) (-5.2765, 0.2857) (-5.2882, 0.2804) (-5.2998, 0.2751) (-5.3115, 0.2697) (-5.3232, 0.2642) (-5.3348, 0.2586) (-5.3465, 0.253) (-5.3581, 0.2473) (-5.3698, 0.2415) (-5.3814, 0.2357) (-5.393, 0.2298) (-5.4047, 0.2238) (-5.4163, 0.2178) (-5.4279, 0.2117) (-5.4395, 0.2055) (-5.451, 0.1993) (-5.4626, 0.193) (-5.4742, 0.1866) (-5.4834, 0.1815) (-5.4903, 0.1776) (-5.4949, 0.175) (-5.4973, 0.1737) knots 0 0 0 0 0 0 0.01428571 0.02857143 0.04285714 0.05714286 0.07142857 0.08571429 0.1 0.11428571 0.12857143 0.14285714 0.15714286 0.17142857 0.18571429 0.2 0.21428571 0.22857143 0.24285714 0.25714286 0.27142857 0.28571429 0.3 0.31428571 0.32857143 0.34285714 0.35714286 0.37142857 0.38571429 0.4 0.41428571 0.42857143 0.44285714 0.45714286 0.47142857 0.48571429 0.5 0.51428571 0.52857143 0.54285714 0.55714286 0.57142857 0.58571429 0.6 0.61428571 0.62857143 0.64285714 0.65714286 0.67142857 0.68571429 0.7 0.71428571 0.72857143 0.74285714 0.75714286 0.77142857 0.78571429 0.8 0.81428571 0.82857143 0.84285714 0.85714286 0.87142857 0.88571429 0.9 0.91428571 0.92857143 0.94285714 0.95714286 0.97142857 0.98571429 1 1 1 1 1 1
  arc A2 (-5.4973, 0.1737) -> (-5.4973, -0.1737) centre (0, 0) ccw
  spline S1 degree 5 poles (-5.4973, -0.1737) (-5.4949, -0.175) (-5.4903, -0.1776) (-5.4834, -0.1815) (-5.4742, -0.1866) (-5.4626, -0.193) (-5.451, -0.1993) (-5.4395, -0.2055) (-5.4279, -0.2117) (-5.4163, -0.2178) (-5.4047, -0.2238) (-5.393, -0.2298) (-5.3814, -0.2357) (-5.3698, -0.2415) (-5.3581, -0.2473) (-5.3465, -0.253) (-5.3348, -0.2586) (-5.3232, -0.2642) (-5.3115, -0.2697) (-5.2998, -0.2751) (-5.2882, -0.2804) (-5.2765, -0.2857) (-5.2648, -0.2909) (-5.2531, -0.296) (-5.2414, -0.3011) (-5.2297, -0.3061) (-5.2179, -0.311) (-5.2062, -0.3158) (-5.1945, -0.3206) (-5.1828, -0.3253) (-5.171, -0.3299) (-5.1593, -0.3344) (-5.1475, -0.3389) (-5.1358, -0.3433) (-5.124, -0.3476) (-5.1123, -0.3518) (-5.1005, -0.3559) (-5.0888, -0.36) (-5.077, -0.364) (-5.0652, -0.3679) (-5.0535, -0.3717) (-5.0417, -0.3754) (-5.0299, -0.3791) (-5.0181, -0.3826) (-5.0064, -0.3861) (-4.9946, -0.3895) (-4.9828, -0.3928) (-4.971, -0.396) (-4.9593, -0.3991) (-4.9475, -0.4022) (-4.9357, -0.4051) (-4.9239, -0.4079) (-4.9122, -0.4106) (-4.9004, -0.4133) (-4.8886, -0.4158) (-4.8769, -0.4182) (-4.8651, -0.4205) (-4.8534, -0.4227) (-4.8416, -0.4248) (-4.8299, -0.4269) (-4.8181, -0.4287) (-4.8064, -0.4304) (-4.7947, -0.432) (-4.7829, -0.4334) (-4.7712, -0.4346) (-4.7595, -0.4357) (-4.7478, -0.4368) (-4.7361, -0.4378) (-4.7245, -0.4386) (-4.7128, -0.4392) (-4.7012, -0.4395) (-4.6919, -0.4393) (-4.6849, -0.439) (-4.6803, -0.4386) (-4.678, -0.4384) knots -1 -1 -1 -1 -1 -1 -0.98571429 -0.97142857 -0.95714286 -0.94285714 -0.92857143 -0.91428571 -0.9 -0.88571429 -0.87142857 -0.85714286 -0.84285714 -0.82857143 -0.81428571 -0.8 -0.78571429 -0.77142857 -0.75714286 -0.74285714 -0.72857143 -0.71428571 -0.7 -0.68571429 -0.67142857 -0.65714286 -0.64285714 -0.62857143 -0.61428571 -0.6 -0.58571429 -0.57142857 -0.55714286 -0.54285714 -0.52857143 -0.51428571 -0.5 -0.48571429 -0.47142857 -0.45714286 -0.44285714 -0.42857143 -0.41428571 -0.4 -0.38571429 -0.37142857 -0.35714286 -0.34285714 -0.32857143 -0.31428571 -0.3 -0.28571429 -0.27142857 -0.25714286 -0.24285714 -0.22857143 -0.21428571 -0.2 -0.18571429 -0.17142857 -0.15714286 -0.14285714 -0.12857143 -0.11428571 -0.1 -0.08571429 -0.07142857 -0.05714286 -0.04285714 -0.02857143 -0.01428571 0 0 0 0 0 0
  line L1 (-4.678, -0.4384) -> (-4.4283, -0.4157)
  arc A3 (-4.3199, -0.5037) -> (-4.4283, -0.4157) centre (-4.4193, -0.5152) ccw
  arc A4 (-4.3199, -0.5037) -> (-4.2641, -0.8559) centre (0, 0) ccw
  arc A5 (-4.34, -0.9731) -> (-4.2641, -0.8559) centre (-4.3622, -0.8756) ccw
  line L2 (-4.34, -0.9731) -> (-4.5845, -1.0286)
  spline S2 degree 5 poles (-4.5845, -1.0286) (-4.5868, -1.0291) (-4.5913, -1.0302) (-4.598, -1.032) (-4.6069, -1.0348) (-4.6179, -1.0386) (-4.6288, -1.0428) (-4.6396, -1.0472) (-4.6504, -1.0517) (-4.6612, -1.0564) (-4.672, -1.061) (-4.6828, -1.0659) (-4.6935, -1.0708) (-4.7042, -1.0759) (-4.7148, -1.0811) (-4.7254, -1.0865) (-4.7359, -1.0921) (-4.7465, -1.0977) (-4.7569, -1.1035) (-4.7674, -1.1093) (-4.7779, -1.1153) (-4.7883, -1.1213) (-4.7987, -1.1274) (-4.809, -1.1336) (-4.8193, -1.14) (-4.8296, -1.1464) (-4.8399, -1.1529) (-4.8501, -1.1595) (-4.8603, -1.1662) (-4.8705, -1.173) (-4.8807, -1.1798) (-4.8908, -1.1868) (-4.9009, -1.1938) (-4.9109, -1.2009) (-4.921, -1.2081) (-4.931, -1.2154) (-4.941, -1.2227) (-4.9509, -1.2301) (-4.9609, -1.2376) (-4.9708, -1.2452) (-4.9806, -1.2528) (-4.9905, -1.2606) (-5.0003, -1.2684) (-5.0101, -1.2762) (-5.0199, -1.2842) (-5.0296, -1.2922) (-5.0393, -1.3003) (-5.049, -1.3084) (-5.0587, -1.3167) (-5.0683, -1.3249) (-5.0779, -1.3333) (-5.0875, -1.3417) (-5.097, -1.3502) (-5.1065, -1.3588) (-5.116, -1.3674) (-5.1255, -1.3761) (-5.1349, -1.3849) (-5.1443, -1.3937) (-5.1537, -1.4026) (-5.163, -1.4115) (-5.1723, -1.4206) (-5.1816, -1.4296) (-5.1909, -1.4388) (-5.2001, -1.448) (-5.2093, -1.4572) (-5.2185, -1.4666) (-5.2276, -1.476) (-5.2367, -1.4854) (-5.2458, -1.4949) (-5.2549, -1.5045) (-5.2639, -1.5141) (-5.2711, -1.5219) (-5.2765, -1.5277) (-5.2801, -1.5316) (-5.2819, -1.5336) knots 0 0 0 0 0 0 0.01428571 0.02857143 0.04285714 0.05714286 0.07142857 0.08571429 0.1 0.11428571 0.12857143 0.14285714 0.15714286 0.17142857 0.18571429 0.2 0.21428571 0.22857143 0.24285714 0.25714286 0.27142857 0.28571429 0.3 0.31428571 0.32857143 0.34285714 0.35714286 0.37142857 0.38571429 0.4 0.41428571 0.42857143 0.44285714 0.45714286 0.47142857 0.48571429 0.5 0.51428571 0.52857143 0.54285714 0.55714286 0.57142857 0.58571429 0.6 0.61428571 0.62857143 0.64285714 0.65714286 0.67142857 0.68571429 0.7 0.71428571 0.72857143 0.74285714 0.75714286 0.77142857 0.78571429 0.8 0.81428571 0.82857143 0.84285714 0.85714286 0.87142857 0.88571429 0.9 0.91428571 0.92857143 0.94285714 0.95714286 0.97142857 0.98571429 1 1 1 1 1 1
  arc A6 (-5.2819, -1.5336) -> (-5.1745, -1.8639) centre (0, 0) ccw
  spline S3 degree 5 poles (-5.1745, -1.8639) (-5.1719, -1.8645) (-5.1667, -1.8655) (-5.1589, -1.8671) (-5.1486, -1.8691) (-5.1356, -1.8716) (-5.1227, -1.874) (-5.1097, -1.8764) (-5.0968, -1.8787) (-5.0839, -1.8809) (-5.071, -1.883) (-5.0581, -1.8851) (-5.0452, -1.8871) (-5.0323, -1.8891) (-5.0195, -1.891) (-5.0066, -1.8928) (-4.9938, -1.8945) (-4.981, -1.8962) (-4.9682, -1.8978) (-4.9554, -1.8994) (-4.9427, -1.9008) (-4.9299, -1.9022) (-4.9172, -1.9036) (-4.9045, -1.9048) (-4.8918, -1.906) (-4.8791, -1.9072) (-4.8664, -1.9082) (-4.8538, -1.9092) (-4.8412, -1.9101) (-4.8286, -1.9109) (-4.816, -1.9117) (-4.8034, -1.9124) (-4.7909, -1.913) (-4.7783, -1.9135) (-4.7658, -1.914) (-4.7533, -1.9144) (-4.7409, -1.9147) (-4.7284, -1.9149) (-4.716, -1.9151) (-4.7036, -1.9151) (-4.6913, -1.9151) (-4.6789, -1.915) (-4.6666, -1.9149) (-4.6543, -1.9146) (-4.642, -1.9143) (-4.6298, -1.9139) (-4.6176, -1.9134) (-4.6054, -1.9128) (-4.5932, -1.9121) (-4.5811, -1.9113) (-4.569, -1.9105) (-4.5569, -1.9095) (-4.5449, -1.9085) (-4.5329, -1.9073) (-4.5209, -1.9061) (-4.509, -1.9047) (-4.4971, -1.9033) (-4.4852, -1.9018) (-4.4734, -1.9002) (-4.4616, -1.8985) (-4.4498, -1.8966) (-4.4381, -1.8946) (-4.4265, -1.8925) (-4.4149, -1.8902) (-4.4034, -1.8877) (-4.3919, -1.8852) (-4.3805, -1.8826) (-4.3691, -1.8799) (-4.3577, -1.8771) (-4.3464, -1.8741) (-4.3353, -1.8707) (-4.3265, -1.8677) (-4.32, -1.8652) (-4.3157, -1.8634) (-4.3135, -1.8625) knots -1 -1 -1 -1 -1 -1 -0.98571429 -0.97142857 -0.95714286 -0.94285714 -0.92857143 -0.91428571 -0.9 -0.88571429 -0.87142857 -0.85714286 -0.84285714 -0.82857143 -0.81428571 -0.8 -0.78571429 -0.77142857 -0.75714286 -0.74285714 -0.72857143 -0.71428571 -0.7 -0.68571429 -0.67142857 -0.65714286 -0.64285714 -0.62857143 -0.61428571 -0.6 -0.58571429 -0.57142857 -0.55714286 -0.54285714 -0.52857143 -0.51428571 -0.5 -0.48571429 -0.47142857 -0.45714286 -0.44285714 -0.42857143 -0.41428571 -0.4 -0.38571429 -0.37142857 -0.35714286 -0.34285714 -0.32857143 -0.31428571 -0.3 -0.28571429 -0.27142857 -0.25714286 -0.24285714 -0.22857143 -0.21428571 -0.2 -0.18571429 -0.17142857 -0.15714286 -0.14285714 -0.12857143 -0.11428571 -0.1 -0.08571429 -0.07142857 -0.05714286 -0.04285714 -0.02857143 -0.01428571 0 0 0 0 0 0
  line L3 (-4.3135, -1.8625) -> (-4.0832, -1.7637)
  arc A7 (-3.9529, -1.814) -> (-4.0832, -1.7637) centre (-4.0437, -1.8557) ccw
  arc A8 (-3.9529, -1.814) -> (-3.791, -2.1317) centre (0, 0) ccw
  arc A9 (-3.8269, -2.2666) -> (-3.791, -2.1317) centre (-3.8781, -2.1807) ccw
  line L4 (-3.8269, -2.2666) -> (-4.0422, -2.395)
  spline S4 degree 5 poles (-4.0422, -2.395) (-4.0442, -2.3962) (-4.0482, -2.3986) (-4.054, -2.4024) (-4.0616, -2.4077) (-4.0709, -2.4148) (-4.08, -2.4221) (-4.0889, -2.4297) (-4.0978, -2.4373) (-4.1067, -2.445) (-4.1155, -2.4528) (-4.1242, -2.4607) (-4.1329, -2.4687) (-4.1415, -2.4769) (-4.1499, -2.4852) (-4.1583, -2.4936) (-4.1667, -2.5021) (-4.1749, -2.5107) (-4.1831, -2.5195) (-4.1913, -2.5282) (-4.1994, -2.5371) (-4.2074, -2.5461) (-4.2154, -2.5551) (-4.2233, -2.5642) (-4.2312, -2.5734) (-4.239, -2.5827) (-4.2467, -2.5921) (-4.2544, -2.6015) (-4.2621, -2.611) (-4.2697, -2.6206) (-4.2772, -2.6303) (-4.2847, -2.64) (-4.2921, -2.6498) (-4.2995, -2.6597) (-4.3068, -2.6696) (-4.3141, -2.6796) (-4.3213, -2.6897) (-4.3285, -2.6998) (-4.3356, -2.71) (-4.3427, -2.7203) (-4.3497, -2.7306) (-4.3567, -2.741) (-4.3636, -2.7515) (-4.3705, -2.762) (-4.3773, -2.7726) (-4.3841, -2.7832) (-4.3909, -2.7939) (-4.3976, -2.8046) (-4.4042, -2.8154) (-4.4108, -2.8263) (-4.4173, -2.8372) (-4.4238, -2.8482) (-4.4303, -2.8592) (-4.4367, -2.8703) (-4.443, -2.8814) (-4.4494, -2.8926) (-4.4556, -2.9039) (-4.4618, -2.9152) (-4.468, -2.9265) (-4.4741, -2.9379) (-4.4802, -2.9494) (-4.4862, -2.9609) (-4.4922, -2.9724) (-4.4981, -2.984) (-4.504, -2.9957) (-4.5099, -3.0074) (-4.5157, -3.0191) (-4.5214, -3.0309) (-4.5271, -3.0428) (-4.5328, -3.0547) (-4.5384, -3.0666) (-4.5428, -3.0762) (-4.5462, -3.0835) (-4.5484, -3.0883) (-4.5495, -3.0907) knots 0 0 0 0 0 0 0.01428571 0.02857143 0.04285714 0.05714286 0.07142857 0.08571429 0.1 0.11428571 0.12857143 0.14285714 0.15714286 0.17142857 0.18571429 0.2 0.21428571 0.22857143 0.24285714 0.25714286 0.27142857 0.28571429 0.3 0.31428571 0.32857143 0.34285714 0.35714286 0.37142857 0.38571429 0.4 0.41428571 0.42857143 0.44285714 0.45714286 0.47142857 0.48571429 0.5 0.51428571 0.52857143 0.54285714 0.55714286 0.57142857 0.58571429 0.6 0.61428571 0.62857143 0.64285714 0.65714286 0.67142857 0.68571429 0.7 0.71428571 0.72857143 0.74285714 0.75714286 0.77142857 0.78571429 0.8 0.81428571 0.82857143 0.84285714 0.85714286 0.87142857 0.88571429 0.9 0.91428571 0.92857143 0.94285714 0.95714286 0.97142857 0.98571429 1 1 1 1 1 1
  arc A10 (-4.5495, -3.0907) -> (-4.3453, -3.3717) centre (0, 0) ccw
  spline S5 degree 5 poles (-4.3453, -3.3717) (-4.3426, -3.3714) (-4.3374, -3.3708) (-4.3295, -3.3699) (-4.319, -3.3686) (-4.3059, -3.367) (-4.2928, -3.3653) (-4.2798, -3.3635) (-4.2668, -3.3617) (-4.2538, -3.3598) (-4.2409, -3.3579) (-4.228, -3.3559) (-4.2151, -3.3538) (-4.2023, -3.3517) (-4.1895, -3.3495) (-4.1767, -3.3473) (-4.164, -3.345) (-4.1513, -3.3426) (-4.1386, -3.3402) (-4.126, -3.3377) (-4.1134, -3.3352) (-4.1008, -3.3326) (-4.0883, -3.3299) (-4.0758, -3.3272) (-4.0634, -3.3244) (-4.051, -3.3215) (-4.0386, -3.3186) (-4.0263, -3.3157) (-4.014, -3.3126) (-4.0017, -3.3095) (-3.9895, -3.3063) (-3.9774, -3.3031) (-3.9652, -3.2998) (-3.9532, -3.2964) (-3.9411, -3.293) (-3.9291, -3.2895) (-3.9172, -3.286) (-3.9053, -3.2823) (-3.8934, -3.2787) (-3.8816, -3.2749) (-3.8698, -3.2711) (-3.8581, -3.2672) (-3.8465, -3.2632) (-3.8348, -3.2592) (-3.8233, -3.255) (-3.8118, -3.2509) (-3.8003, -3.2466) (-3.7889, -3.2423) (-3.7775, -3.2379) (-3.7662, -3.2334) (-3.755, -3.2289) (-3.7438, -3.2242) (-3.7327, -3.2195) (-3.7216, -3.2147) (-3.7106, -3.2098) (-3.6997, -3.2049) (-3.6888, -3.1998) (-3.678, -3.1947) (-3.6672, -3.1895) (-3.6565, -3.1843) (-3.6459, -3.1789) (-3.6354, -3.1734) (-3.625, -3.1677) (-3.6148, -3.1619) (-3.6045, -3.1561) (-3.5944, -3.1501) (-3.5843, -3.1441) (-3.5743, -3.138) (-3.5644, -3.1318) (-3.5546, -3.1254) (-3.545, -3.1188) (-3.5376, -3.1132) (-3.5321, -3.1089) (-3.5286, -3.1058) (-3.5269, -3.1043) knots -1 -1 -1 -1 -1 -1 -0.98571429 -0.97142857 -0.95714286 -0.94285714 -0.92857143 -0.91428571 -0.9 -0.88571429 -0.87142857 -0.85714286 -0.84285714 -0.82857143 -0.81428571 -0.8 -0.78571429 -0.77142857 -0.75714286 -0.74285714 -0.72857143 -0.71428571 -0.7 -0.68571429 -0.67142857 -0.65714286 -0.64285714 -0.62857143 -0.61428571 -0.6 -0.58571429 -0.57142857 -0.55714286 -0.54285714 -0.52857143 -0.51428571 -0.5 -0.48571429 -0.47142857 -0.45714286 -0.44285714 -0.42857143 -0.41428571 -0.4 -0.38571429 -0.37142857 -0.35714286 -0.34285714 -0.32857143 -0.31428571 -0.3 -0.28571429 -0.27142857 -0.25714286 -0.24285714 -0.22857143 -0.21428571 -0.2 -0.18571429 -0.17142857 -0.15714286 -0.14285714 -0.12857143 -0.11428571 -0.1 -0.08571429 -0.07142857 -0.05714286 -0.04285714 -0.02857143 -0.01428571 0 0 0 0 0 0
  line L5 (-3.5269, -3.1043) -> (-3.3383, -2.9392)
  arc A11 (-3.1989, -2.9467) -> (-3.3383, -2.9392) centre (-3.2724, -3.0144) ccw
  arc A12 (-3.1989, -2.9467) -> (-2.9467, -3.1989) centre (0, 0) ccw
  arc A13 (-2.9392, -3.3383) -> (-2.9467, -3.1989) centre (-3.0144, -3.2724) ccw
  line L6 (-2.9392, -3.3383) -> (-3.1043, -3.5269)
  spline S6 degree 5 poles (-3.1043, -3.5269) (-3.1058, -3.5286) (-3.1089, -3.5321) (-3.1132, -3.5376) (-3.1188, -3.545) (-3.1254, -3.5546) (-3.1318, -3.5644) (-3.138, -3.5743) (-3.1441, -3.5843) (-3.1501, -3.5944) (-3.1561, -3.6045) (-3.1619, -3.6148) (-3.1677, -3.625) (-3.1734, -3.6354) (-3.1789, -3.6459) (-3.1843, -3.6565) (-3.1895, -3.6672) (-3.1947, -3.678) (-3.1998, -3.6888) (-3.2049, -3.6997) (-3.2098, -3.7106) (-3.2147, -3.7216) (-3.2195, -3.7327) (-3.2242, -3.7438) (-3.2289, -3.755) (-3.2334, -3.7662) (-3.2379, -3.7775) (-3.2423, -3.7889) (-3.2466, -3.8003) (-3.2509, -3.8118) (-3.255, -3.8233) (-3.2592, -3.8348) (-3.2632, -3.8465) (-3.2672, -3.8581) (-3.2711, -3.8698) (-3.2749, -3.8816) (-3.2787, -3.8934) (-3.2823, -3.9053) (-3.286, -3.9172) (-3.2895, -3.9291) (-3.293, -3.9411) (-3.2964, -3.9532) (-3.2998, -3.9652) (-3.3031, -3.9774) (-3.3063, -3.9895) (-3.3095, -4.0017) (-3.3126, -4.014) (-3.3157, -4.0263) (-3.3186, -4.0386) (-3.3215, -4.051) (-3.3244, -4.0634) (-3.3272, -4.0758) (-3.3299, -4.0883) (-3.3326, -4.1008) (-3.3352, -4.1134) (-3.3377, -4.126) (-3.3402, -4.1386) (-3.3426, -4.1513) (-3.345, -4.164) (-3.3473, -4.1767) (-3.3495, -4.1895) (-3.3517, -4.2023) (-3.3538, -4.2151) (-3.3559, -4.228) (-3.3579, -4.2409) (-3.3598, -4.2538) (-3.3617, -4.2668) (-3.3635, -4.2798) (-3.3653, -4.2928) (-3.367, -4.3059) (-3.3686, -4.319) (-3.3699, -4.3295) (-3.3708, -4.3374) (-3.3714, -4.3426) (-3.3717, -4.3453) knots 0 0 0 0 0 0 0.01428571 0.02857143 0.04285714 0.05714286 0.07142857 0.08571429 0.1 0.11428571 0.12857143 0.14285714 0.15714286 0.17142857 0.18571429 0.2 0.21428571 0.22857143 0.24285714 0.25714286 0.27142857 0.28571429 0.3 0.31428571 0.32857143 0.34285714 0.35714286 0.37142857 0.38571429 0.4 0.41428571 0.42857143 0.44285714 0.45714286 0.47142857 0.48571429 0.5 0.51428571 0.52857143 0.54285714 0.55714286 0.57142857 0.58571429 0.6 0.61428571 0.62857143 0.64285714 0.65714286 0.67142857 0.68571429 0.7 0.71428571 0.72857143 0.74285714 0.75714286 0.77142857 0.78571429 0.8 0.81428571 0.82857143 0.84285714 0.85714286 0.87142857 0.88571429 0.9 0.91428571 0.92857143 0.94285714 0.95714286 0.97142857 0.98571429 1 1 1 1 1 1
  arc A14 (-3.3717, -4.3453) -> (-3.0907, -4.5495) centre (0, 0) ccw
  spline S7 degree 5 poles (-3.0907, -4.5495) (-3.0883, -4.5484) (-3.0835, -4.5462) (-3.0762, -4.5428) (-3.0666, -4.5384) (-3.0547, -4.5328) (-3.0428, -4.5271) (-3.0309, -4.5214) (-3.0191, -4.5157) (-3.0074, -4.5099) (-2.9957, -4.504) (-2.984, -4.4981) (-2.9724, -4.4922) (-2.9609, -4.4862) (-2.9494, -4.4802) (-2.9379, -4.4741) (-2.9265, -4.468) (-2.9152, -4.4618) (-2.9039, -4.4556) (-2.8926, -4.4494) (-2.8814, -4.443) (-2.8703, -4.4367) (-2.8592, -4.4303) (-2.8482, -4.4238) (-2.8372, -4.4173) (-2.8263, -4.4108) (-2.8154, -4.4042) (-2.8046, -4.3976) (-2.7939, -4.3909) (-2.7832, -4.3841) (-2.7726, -4.3773) (-2.762, -4.3705) (-2.7515, -4.3636) (-2.741, -4.3567) (-2.7306, -4.3497) (-2.7203, -4.3427) (-2.71, -4.3356) (-2.6998, -4.3285) (-2.6897, -4.3213) (-2.6796, -4.3141) (-2.6696, -4.3068) (-2.6597, -4.2995) (-2.6498, -4.2921) (-2.64, -4.2847) (-2.6303, -4.2772) (-2.6206, -4.2697) (-2.611, -4.2621) (-2.6015, -4.2544) (-2.5921, -4.2467) (-2.5827, -4.239) (-2.5734, -4.2312) (-2.5642, -4.2233) (-2.5551, -4.2154) (-2.5461, -4.2074) (-2.5371, -4.1994) (-2.5282, -4.1913) (-2.5195, -4.1831) (-2.5107, -4.1749) (-2.5021, -4.1667) (-2.4936, -4.1583) (-2.4852, -4.1499) (-2.4769, -4.1415) (-2.4687, -4.1329) (-2.4607, -4.1242) (-2.4528, -4.1155) (-2.445, -4.1067) (-2.4373, -4.0978) (-2.4297, -4.0889) (-2.4221, -4.08) (-2.4148, -4.0709) (-2.4077, -4.0616) (-2.4024, -4.054) (-2.3986, -4.0482) (-2.3962, -4.0442) (-2.395, -4.0422) knots -1 -1 -1 -1 -1 -1 -0.98571429 -0.97142857 -0.95714286 -0.94285714 -0.92857143 -0.91428571 -0.9 -0.88571429 -0.87142857 -0.85714286 -0.84285714 -0.82857143 -0.81428571 -0.8 -0.78571429 -0.77142857 -0.75714286 -0.74285714 -0.72857143 -0.71428571 -0.7 -0.68571429 -0.67142857 -0.65714286 -0.64285714 -0.62857143 -0.61428571 -0.6 -0.58571429 -0.57142857 -0.55714286 -0.54285714 -0.52857143 -0.51428571 -0.5 -0.48571429 -0.47142857 -0.45714286 -0.44285714 -0.42857143 -0.41428571 -0.4 -0.38571429 -0.37142857 -0.35714286 -0.34285714 -0.32857143 -0.31428571 -0.3 -0.28571429 -0.27142857 -0.25714286 -0.24285714 -0.22857143 -0.21428571 -0.2 -0.18571429 -0.17142857 -0.15714286 -0.14285714 -0.12857143 -0.11428571 -0.1 -0.08571429 -0.07142857 -0.05714286 -0.04285714 -0.02857143 -0.01428571 0 0 0 0 0 0
  line L7 (-2.395, -4.0422) -> (-2.2666, -3.8269)
  arc A15 (-2.1317, -3.791) -> (-2.2666, -3.8269) centre (-2.1807, -3.8781) ccw
  arc A16 (-2.1317, -3.791) -> (-1.814, -3.9529) centre (0, 0) ccw
  arc A17 (-1.7637, -4.0832) -> (-1.814, -3.9529) centre (-1.8557, -4.0437) ccw
  line L8 (-1.7637, -4.0832) -> (-1.8625, -4.3135)